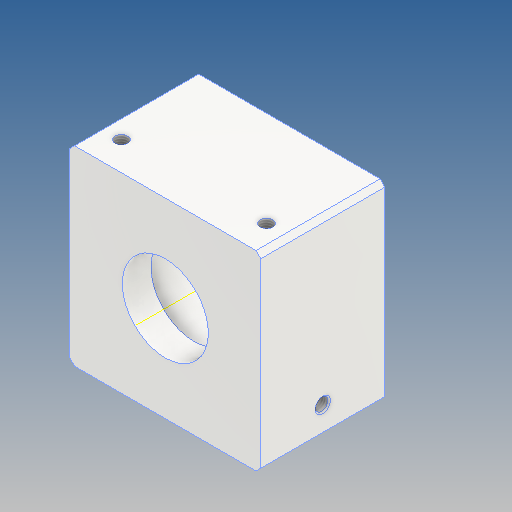
# Autodesk Inventor part: 200-10-ROCKER-BEARING-01
Saved by Autodesk Inventor 2018.2 (Build 222227000, 227)
## iProperties
Manager: feesmrt
Company: FRANCOR
Created: 2017-10-25
Part Number: 200-10-ROCKER-BEARING-01
Material: Aluminium 6061
Document SubType Name: Modeling
Designer: feesmrt
Density: 2.7 g/cm^3
Appearance: Aluminium - flach
Project: Rescue Robot
Description: Rocker Bearing Housing
Engineer: feesmrt
Authority: feesmrt
Stock Number: 200-10-ROCKER-BEARING-01
Mass: 1082.5 g
Surface Area: 586.282 cm^2
Volume: 400.925 cm^3
Cost Center: -
Author: feesmrt
Title: Rocker Housing
Subject: Rescue Robot
Revision Number: 1
Autodesk Inventor part; units mm, degrees
ref_plane "YZ Plane" through (0, 0, 0) normal (1, 0, 0) x (0, 1, 0)
ref_plane "XZ Plane" through (0, 0, 0) normal (0, 1, 0) x (-1, 0, 0)
ref_plane "XY Plane" through (0, 0, 0) normal (0, 0, 1) x (1, 0, 0)
sketch "Skizze1" plane through (0, 0, 0) normal (0, 1, 0) x (-1, 0, 0)
  line L0 (0, -50) -> (-50, -50)
  line L1 (-50, -50) -> (-50, 50)
  line L2 (-50, 50) -> (0, 50)
  line L3 (0, -50) -> (50, -50)
  line L4 (50, -50) -> (50, 50)
  line L5 (50, 50) -> (0, 50)
  line L6 (-122.5, 0) -> (122.5, 0) construction
  line L7 (0, -77.2) -> (0, 113.2) construction
  dimension "d1" = 100
  dimension "d3" = 100
  constraints: 12 end point, 3 horizontal, 1 parallel, 1 point on line, 1 vertical, 2 other
  measures "d1" distance between parallel lines of L0 L2
  measures "d3" distance between parallel lines of L1 L4
extrude "Grundkoerper" add sketch "Skizze1" along normal mid plane 65
sketch "Skizze2" plane through (0, -32.5, 0) normal (0, -1, 0) x (1, 0, 0)
  line L0 (-50, -50) -> (50, -50) projected
  line L1 (50, 50) -> (-50, 50) projected
  point P0 (0, 0)
  point P1 (0, 0)
  point P2 (-87.5, 0)
  point P3 (87.5, 0)
  dimension "d8" = 0
  constraints: 1 other
  measures "d8" distance of point (0, 0) point (0, 0)
sketch "Skizze3" plane through (0, 0, 0) normal (1, 0, 0) x (0, 1, 0)
  line L0 (49, 0) -> (-49, 0) construction
  line L1 (-32.5, 50) -> (-32.5, -50) construction
  line L2 (32.5, -50) -> (32.5, 50) construction
  line L3 (17.5, 36) -> (-12.5, 36)
  line L4 (-12.5, 36) -> (-12.5, 31)
  line L5 (-17.5, 22.5) -> (-32.5, 22.5)
  line L6 (-32.5, -50) -> (-32.5, 50) projected
  line L7 (-32.5, 22.5) -> (-32.5, 0)
  line L8 (-32.5, 0) -> (32.5, 0)
  line L9 (32.5, 0) -> (32.5, 37.5)
  line L10 (-12.5, 31) -> (-17.5, 31)
  line L11 (-17.5, 31) -> (-17.5, 22.5)
  line L12 (17.5, 36) -> (17.5, 37.5)
  line L13 (17.5, 37.5) -> (32.5, 37.5)
  point P0 (0, 0)
  dimension "d9" = 45
  dimension "d10" = 72
  dimension "d11" = 45
  dimension "d33" = 5
  dimension "d34" = 62
  dimension "d160" = 75
  dimension "d161" = 30
  constraints: 20 end point, 6 perpendicular, 4 point on line, 2 horizontal, 2 midpoint
  measures "d9" distance between parallel lines of L2 L4
  measures "d10" diameter of L3 L0
  measures "d11" diameter of L5 L0
  measures "d33" distance of L4.end L10.end
  measures "d34" diameter of L10 L0
  measures "d160" diameter of L13 L0
  measures "d161" distance between parallel lines of L4 L12
revolve "Lagersitz" cut sketch "Skizze3" angle 360 about axis through (0, -32.5, 0) along (0, -1, 0)
sketch "Skizze_Lagersitz" plane through (0, 0, 0) normal (1, 0, 0) x (0, 1, 0)
  line L0 (-12.5, 36) -> (17.5, 36) projected
  line L1 (-12.5, -36) -> (-12.5, 36) projected
  line L2 (-17.5, 31) -> (-12.5, 31) projected
  line L3 (-17.5, -31) -> (-17.5, 31) projected
  line L4 (-32.5, 22.5) -> (-17.5, 22.5) projected
  line L5 (-32.5, -22.5) -> (-17.5, -22.5) projected
  line L6 (-17.5, -31) -> (-12.5, -31) projected
  line L7 (-12.5, -36) -> (17.5, -36) projected
  line L8 (32.5, 50) -> (32.5, -50) projected
  line L9 (30, -50) -> (30, 0) projected
  line L10 (-32.5, -22.5) -> (-32.5, 22.5) projected
  line L11 (-32.5, 50) -> (-32.5, -50) projected
  line L12 (-32.5, -50) -> (-32.5, 50) projected
  line L13 (-12.5, -36) -> (-12.5, 36) projected
  line L14 (17.5, -37.5) -> (17.5, 37.5) projected
  line L15 (17.5, 37.5) -> (32.5, 37.5) projected
  point P0 (0, 0)
  point P1 (30, 86)
  point P2 (30, 14)
  point P3 (-30, 32)
  point P4 (-30, 68)
  point P5 (32.5, 36)
  point P6 (32.5, -36)
  constraints: 2 other
sketch "Skizze5" plane through (0, 32.5, 0) normal (0, 1, 0) x (1, 0, 0)
  line L0 (0, 77.2) -> (0, -113.2) construction
  circle A0 centre (0, 0) radius 42.5 construction
  line L1 (122.5, 0) -> (-122.5, 0) construction
  point P0 (42.5, 0)
  point P1 (21.25, 36.8061)
  point P2 (-21.25, 36.8061)
  point P3 (-42.5, 0)
  point P4 (-21.25, -36.8061)
  point P5 (21.25, -36.8061)
  dimension "d167" = 85
  dimension "d170" = 360
  constraints: 2 coincident, 1 horizontal alignment, 1 point on line, 9 other
hole "M5x10_Deckel" at (42.5, 32.5, 0) at (21.25, 32.5, -36.8061) at (-21.25, 32.5, -36.8061) at (-42.5, 32.5, 0) at (-21.25, 32.5, 36.8061) at (21.25, 32.5, 36.8061) direction (0, -1, 0) diameter 4.134 depth 14.2 tip angle 118 countersink diameter 5 countersink angle 90 thread size "M5x0.8" class "6H" standard "ISO Metric profile"
sketch "Skizze9" plane through (50, -32.5, -50) normal (1, 0, 0) x (0, 0, -1)
  line L0 (-50, 81.5) -> (-50, -16.5) construction
  line L1 (0, 65) -> (0, 0) construction
  line L2 (-100, 65) -> (0, 65) construction
  line L3 (0, 0) -> (-100, 0) construction
  line L4 (-163.2, 32.5) -> (27.2, 32.5) construction
  point P0 (-50, 32.5)
  point P1 (-15, 32.5)
  dimension "d94" = 50
  dimension "d95" = 15
  constraints: 1 point on line, 1 other
  measures "d94" distance of the line from the sketch origin of L0
hole "M8x16_Seite" at (50, 0, -35) direction (-1, 0, 0) diameter 6.647 depth 22.2 tip angle 118 countersink diameter 8 countersink angle 90 thread size "M8x1.25" class "6H" standard "ISO Metric profile"
mirror "M8x16_Seite_Spiegel" about plane through (0, 0, 0) normal (1, 0, 0) of "M8x16_Seite"
sketch "Skizze16" plane through (50, 32.5, -50) normal (0, 0, -1) x (-1, 0, 0)
  line L0 (50, -78) -> (50, 13) construction
  line L1 (100, -65) -> (0, -65) construction
  line L2 (100, 0) -> (100, -65) projected
  point P0 (50, -32.5)
  point P1 (88, -50)
  point P2 (12, -50)
  dimension "d181" = 76
  dimension "d182" = 15
  dimension "d183" = 12
  constraints: 1 symmetric about line
  measures "d181" distance of point (12, -50) point (88, -50)
  measures "d182" distance from line of L1 point (88, -50)
  measures "d183" distance from line of point (88, -50) L2
hole "M8x16_Boden" at (-38, -17.5, -50) at (38, -17.5, -50) direction (0, 0, 1) diameter 6.647 depth 22.2 tip angle 118 thread size "M8x1.25" class "6H" standard "ISO Metric profile"
mirror "M8x16_Deckel" about plane through (0, 0, 0) normal (0, 0, 1) of "M8x16_Boden"
chamfer "Fase_Lagersitz" distance 0.25 angle 45 1 edges at (0, -12.5, -31)
chamfer "Fase_Deckel" distance 1 angle 45 1 edges at (0, 32.5, -37.5)
chamfer "Fase_Allgemein" distance 2.5 angle 45 4 edges at (50, 0, 50) (-50, 0, 50) (50, 0, -50) (-50, 0, -50)
